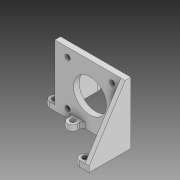
# Autodesk Inventor part: PitchMotorBracket
Saved by Autodesk Inventor 2020 (Build 240168000, 168)
## iProperties
Created: 2020-09-19
Part Number: PitchMotorBracket
Material: Generic
Document SubType Name: Modeling
Designer: DDeGo
Density: 1 g/cm^3
Appearance: Default
Author: DDeGo
Autodesk Inventor part; units mm, degrees
ref_plane "YZ Plane" through (0, 0, 0) normal (1, 0, 0) x (0, 1, 0)
ref_plane "XZ Plane" through (0, 0, 0) normal (0, 1, 0) x (-1, 0, 0)
ref_plane "XY Plane" through (0, 0, 0) normal (0, 0, 1) x (1, 0, 0)
sketch "Sketch1" plane through (0, 0, 0) normal (0, 0, 1) x (1, 0, 0)
  line L0 (-15.5, 15.5) -> (15.5, 15.5) construction
  line L1 (15.5, 15.5) -> (15.5, -15.5) construction
  line L2 (15.5, -15.5) -> (-15.5, -15.5) construction
  line L3 (-15.5, -15.5) -> (-15.5, 15.5) construction
  line L4 (-15.5, 15.5) -> (15.5, -15.5) construction
  line L5 (15.5, 15.5) -> (-15.5, -15.5) construction
  circle A0 centre (0, 0) radius 11.5
  circle A1 centre (15.5, 15.5) radius 1.75
  circle A2 centre (15.5, -15.5) radius 1.75
  circle A3 centre (-15.5, -15.5) radius 1.75
  circle A4 centre (-15.5, 15.5) radius 1.75
  line L6 (-21.5, -21.5) -> (21.5, -21.5)
  line L7 (21.5, -21.5) -> (21.5, 21.5)
  line L8 (21.5, 21.5) -> (-21.5, 21.5)
  line L9 (-21.5, 21.5) -> (-21.5, -21.5)
  line L10 (-21.5, -21.5) -> (21.5, 21.5) construction
  line L11 (21.5, -21.5) -> (-21.5, 21.5) construction
  dimension "d0" = 23
  dimension "d1" = 3.5
  dimension "d2" = 31
  dimension "d3" = 31
  dimension "d4" = 43
  constraints: 24 end point, 6 coincident, 5 centre point, 4 midpoint, 4 parallel, 3 equal radius, 2 horizontal, 2 perpendicular, 1 point on line
  measures "d0" diameter of A0
  measures "d1" diameter of A4
  measures "d2" distance of L0.start L1.start
  measures "d3" distance of L2.end L0.start
  measures "d4" distance of L6.end L7.end
extrude "Extrusion1" add sketch "Sketch1" against normal mid plane 4
sketch "Sketch2" plane through (-21.5, -21.5, -2) normal (-1, 0, 0) x (0, 0, 1)
  line L0 (0, 43) -> (4, 43) projected
  line L1 (0, 0) -> (0, 43) projected
  line L2 (0, 0) -> (4, 0) projected
  line L3 (4, 43) -> (4, 0) projected
  line L4 (0, 43) -> (4, 43) projected
  line L5 (0, 43) -> (-28, 4)
  line L6 (-28, 4) -> (-28, 0)
  line L7 (0, 43) -> (0, 0) projected
  line L8 (-28, 0) -> (0, 0)
  point P0 (2, 21.5)
  dimension "d7" = 28
  dimension "d8" = 4
  constraints: 6 end point, 2 perpendicular
  measures "d7" distance of L6.end L1.start
  measures "d8" distance of L5.end L6.end
extrude "Extrusion2" add sketch "Sketch2" along normal blind 3
sketch "Sketch3" plane through (21.5, -21.5, -2) normal (1, 0, 0) x (0, 0, -1)
  line L0 (-4, 0) -> (0, 0) projected
  line L1 (0, 43) -> (0, 0) projected
  line L2 (0, 43) -> (-4, 43) projected
  line L3 (-4, 0) -> (-4, 43) projected
  line L4 (-4, 0) -> (-4, 43) projected
  line L5 (-4, 43) -> (-29, 4)
  line L6 (-29, 4) -> (-29, 0)
  line L7 (-29, 0) -> (-4, 0)
  point P0 (-2, 21.5)
  dimension "d11" = 4
  dimension "d12" = 25
  constraints: 6 end point, 1 parallel, 1 perpendicular
  measures "d11" distance of L5.end L6.end
  measures "d12" distance of L6.end L0.start
extrude "Extrusion3" add sketch "Sketch3" along normal blind 3
sketch "Sketch4" plane through (-21.5, -21.5, -30) normal (0, -1, 0) x (1, 0, 0)
  arc A0 (39.5, 57) -> (39.5, 50) centre (39.5, 53.5) ccw
  line L0 (43, 32) -> (43, 57) projected
  line L1 (43, 57) -> (39.5, 57)
  line L2 (39.5, 50) -> (43, 50)
  line L3 (39.5, 50) -> (39.5, 57) construction
  circle A1 centre (39.5, 53.5) radius 1.75
  arc A2 (-6.5, 32) -> (-6.5, 25) centre (-6.5, 28.5) ccw
  line L4 (-3, 32) -> (-6.5, 32)
  line L5 (-6.5, 25) -> (-3, 25)
  line L6 (-6.5, 25) -> (-6.5, 32) construction
  circle A3 centre (-6.5, 28.5) radius 1.75
  arc A4 (-6.5, 7) -> (-6.5, 0) centre (-6.5, 3.5) ccw
  line L7 (-3, 7) -> (-6.5, 7)
  line L8 (-6.5, 0) -> (-3, 0)
  line L9 (-6.5, 0) -> (-6.5, 7) construction
  circle A5 centre (-6.5, 3.5) radius 1.75
  line L10 (-3, 0) -> (-3, 32) projected
  arc A6 (16.5, 35.5) -> (9.5, 35.5) centre (13, 35.5) ccw
  line L11 (16.5, 32) -> (16.5, 35.5)
  line L12 (9.5, 35.5) -> (9.5, 32)
  line L13 (9.5, 35.5) -> (16.5, 35.5) construction
  circle A7 centre (13, 35.5) radius 1.75
  line L14 (43, 32) -> (-3, 32) projected
  line L15 (0, 28) -> (46, 28) projected
  line L16 (46, 32) -> (46, 57) projected
  point P0 (21.5, 30)
  dimension "d15" = 3.5
  dimension "d16" = 3.5
  dimension "d19" = 3.5
  dimension "d20" = 3.5
  dimension "d21" = 3.5
  dimension "d22" = 3.5
  dimension "d23" = 3.5
  dimension "d24" = 3.5
  dimension "d25" = 16
  dimension "d27" = 25.5
  dimension "d28" = 6.5
  dimension "d31" = 26.5
  dimension "d32" = 19.5
  dimension "d33" = 18
  dimension "d34" = 7
  dimension "d35" = 25
  constraints: 24 end point, 12 tangent, 8 centre point, 8 point on circle, 5 point on line, 4 coincident, 4 perpendicular, 3 horizontal, 1 vertical
  measures "d15" diameter of A1
  measures "d16" radius of A0
  measures "d19" diameter of A3
  measures "d20" radius of A2
  measures "d21" diameter of A5
  measures "d22" radius of A4
  measures "d23" diameter of A7
  measures "d24" radius of A6
  measures "d25" horizontal distance of L4.start A6.centre
  measures "d27" distance from line of L15 A0.centre
  measures "d28" distance from line of A0.centre L16
  measures "d31" horizontal distance of A6.centre A0.centre
  measures "d32" horizontal distance of A2.centre A6.centre
  measures "d33" vertical distance of A0.centre A6.centre
  measures "d34" vertical distance of A2.centre A6.centre
  measures "d35" distance of A4.centre A2.centre
extrude "Extrusion4" add sketch "Sketch4" against normal blind 4
fillet "Fillet1" radius 2 5 edges at (-24.5, -19.5, -23) (-12, -19.5, 2) (-24.5, -19.5, -5) (-5, -19.5, 2) (21.5, -19.5, 20)
fillet "Fillet2" radius 5 1 edges at (-21.5, -19.5, -30)
body "Solid1"
